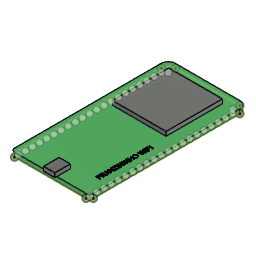
FRANZININHO_WIFI v4 (Autodesk Fusion 360 design; units mm, degrees)
Autodesk Fusion 360 part; units mm, degrees
sketch "Esboço1" plane through (0, 0, 0) normal (0, 1, 0) x (1, 0, 0)
sketch "Esboço2" plane through (0, 0, 0) normal (0, 0, 1) x (1, 0, 0)
  line L0 (2, 52.07) -> (1.27, 52.07)
  line L1 (2, 52.07) -> (24.13, 52.07)
  arc A0 (1.27, 52.07) -> (-1.3, 49.5) centre (1.27, 49.5) ccw
  arc A1 (26.6534, 49.5421) -> (24.13, 52.07) centre (24.13, 49.5466) ccw
  arc A2 (-1.27, -2.55) -> (0, -3.8) centre (-0.01, -2.54) ccw
  arc A3 (25.4, -3.8) -> (26.67, -2.54) centre (25.4137, -2.5438) ccw
  line L2 (0, -3.8) -> (0.5392, -3.8)
  line L3 (0.5392, -3.8) -> (25.4, -3.8)
  line L4 (-1.3, 49.5) -> (-1.27, -2.55)
  line L5 (26.6534, 49.5421) -> (26.67, -2.54)
  constraint horizontal L0
  constraint parallel L0 L1
  constraint tangent L0 A0
  constraint tangent L1 A1
  constraint horizontal L2
  constraint parallel L2 L3
extrude "Extrusão1" add sketch "Esboço2" along normal blind 1.5
sketch "Esboço3" plane through (0, 0, 1.5) normal (0, 0, 1) x (-1, 0, 0)
  line L0 (-24.13, -52.07) -> (-1.27, -52.07)
  arc A0 (-1.27, -52.07) -> (1.3, -49.5) centre (-1.27, -49.5) ccw
  line L1 (1.3, -49.5) -> (1.27, 2.55)
  arc A1 (1.27, 2.55) -> (0, 3.8) centre (0.01, 2.54) ccw
  line L2 (0, 3.8) -> (-25.4, 3.8)
  arc A2 (-25.4, 3.8) -> (-26.67, 2.54) centre (-25.4137, 2.5438) ccw
  line L3 (-26.67, 2.54) -> (-26.6534, -49.5421)
  arc A3 (-26.6534, -49.5421) -> (-24.13, -52.07) centre (-24.13, -49.5466) ccw
  circle A4 centre (0.0063, -48.2369) radius 0.25
  dimension "d3" = 0.5
  measures "d3" diameter of A4
extrude "Extrusão2" add sketch "Esboço3" along normal blind 0.3 contours A4
delete_face "Excluir face1" 1 faces at (-0.2514, 48.2864, 1.7)
sketch "Esboço4" plane through (0, 0, 1.5) normal (0, 0, 1) x (-1, 0, 0)
  line L0 (-24.13, -52.07) -> (-1.27, -52.07)
  arc A0 (-1.27, -52.07) -> (1.3, -49.5) centre (-1.27, -49.5) ccw
  line L1 (1.3, -49.5) -> (1.27, 2.55)
  arc A1 (1.27, 2.55) -> (0, 3.8) centre (0.01, 2.54) ccw
  line L2 (0, 3.8) -> (-25.4, 3.8)
  arc A2 (-25.4, 3.8) -> (-26.67, 2.54) centre (-25.4137, 2.5438) ccw
  line L3 (-26.67, 2.54) -> (-26.6534, -49.5421)
  arc A3 (-26.6534, -49.5421) -> (-24.13, -52.07) centre (-24.13, -49.5466) ccw
  line L4 (-3, -48) -> (-22, -48)
  line L5 (-22, -48) -> (-22, -28)
  line L6 (-22, -28) -> (-3, -28)
  line L7 (-3, -28) -> (-3, -48)
  constraint horizontal L4
  constraint vertical L5
  constraint horizontal L6
  constraint vertical L7
extrude "Extrusão3" add sketch "Esboço4" along normal blind 1.5 contours L4 L5 L6 L7
sketch "Esboço5" plane through (0, 0, 1.5) normal (0, 0, 1) x (-1, 0, 0)
  line L0 (-3, -28) -> (-3, -48)
  line L1 (-3, -48) -> (-22, -48)
  line L2 (-22, -48) -> (-22, -28)
  line L3 (-22, -28) -> (-3, -28)
  line L4 (-24.13, -52.07) -> (-1.27, -52.07)
  arc A0 (-1.27, -52.07) -> (1.3, -49.5) centre (-1.27, -49.5) ccw
  line L5 (1.3, -49.5) -> (1.27, 2.55)
  arc A1 (1.27, 2.55) -> (0, 3.8) centre (0.01, 2.54) ccw
  line L6 (0, 3.8) -> (-25.4, 3.8)
  arc A2 (-25.4, 3.8) -> (-26.67, 2.54) centre (-25.4137, 2.5438) ccw
  line L7 (-26.67, 2.54) -> (-26.6534, -49.5421)
  arc A3 (-26.6534, -49.5421) -> (-24.13, -52.07) centre (-24.13, -49.5466) ccw
  line L8 (-11, -1) -> (-15, -1)
  line L9 (-15, -1) -> (-15, 3.8)
  line L10 (-15, 3.8) -> (-11, 3.8)
  line L11 (-11, 3.8) -> (-11, -1)
  constraint horizontal L8
  constraint vertical L9
  constraint horizontal L10
  constraint vertical L11
  constraint coincident L6 L9.end
extrude "Extrusão4" add sketch "Esboço5" along normal blind 1.5 contours L6 L8 L9 L10 L11
sketch "Esboço6" plane through (0, 0, 0) normal (0, 0, 1) x (1, 0, 0)
sketch "Esboço7" plane through (0, 0, 0) normal (0, 0, 1) x (1, 0, 0)
sketch "Esboço8" plane through (0, 0, 0) normal (0, 1, 0) x (1, 0, 0)
  line L0 (11, -1.5) -> (11.1, -1.5)
  line L1 (11.1, -1.5) -> (15, -1.5)
  line L2 (15, -1.5) -> (15, -3)
  line L3 (15, -3) -> (11, -3)
  line L4 (11, -3) -> (11, -1.5)
  constraint horizontal L0
  constraint parallel L0 L1
  constraint perpendicular L1 L2
  constraint perpendicular L2 L3
  constraint perpendicular L0 L4
extrude "Extrusão5" add sketch "Esboço8" against normal blind 4.5
sketch "Esboço9" plane through (0, 0, 1.5) normal (0, 0, 1) x (-1, 0, 0)
  line L0 (-15, -1) -> (-15, 3.8)
  line L1 (-15, 3.8) -> (-25.4, 3.8)
  arc A0 (-25.4, 3.8) -> (-26.67, 2.54) centre (-25.4137, 2.5438) ccw
  line L2 (-26.67, 2.54) -> (-26.6534, -49.5421)
  arc A1 (-26.6534, -49.5421) -> (-24.13, -52.07) centre (-24.13, -49.5466) ccw
  line L3 (-24.13, -52.07) -> (-1.27, -52.07)
  arc A2 (-1.27, -52.07) -> (1.3, -49.5) centre (-1.27, -49.5) ccw
  line L4 (1.3, -49.5) -> (1.27, 2.55)
  arc A3 (1.27, 2.55) -> (0, 3.8) centre (0.01, 2.54) ccw
  line L5 (0, 3.8) -> (-11, 3.8)
  line L6 (-11, 3.8) -> (-11, -1)
  line L7 (-11, -1) -> (-15, -1)
  line L8 (-3, -28) -> (-3, -48)
  line L9 (-3, -48) -> (-22, -48)
  line L10 (-22, -48) -> (-22, -28)
  line L11 (-22, -28) -> (-3, -28)
sketch "Esboço10" plane through (0, 0, 1.5) normal (0, 0, 1) x (-1, 0, 0)
  line L0 (-25, 0) -> (-25, -25) construction
  line L1 (-25, -25) -> (-22, -25) construction
  line L2 (-22, -25) -> (-22, 0) construction
  line L3 (-22, 0) -> (-25, 0) construction
  dimension "d13" = 1.5
  text T0 "FRANZININHO WIFI" font "Arial" height 1.5 align centre top in box 25 x 3 at (-25, 0) x (0, -1) y (1, 0) spacing 1 kerned
extrude "Extrusão6" add sketch "Esboço10" along normal blind 0.1 text T0
